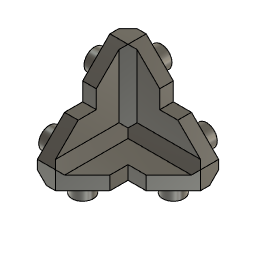
Frame_Corners v4 (Autodesk Fusion 360 design; units mm, degrees)
Autodesk Fusion 360 part; units mm, degrees
sketch "Sketch1" plane through (0, 0, 0) normal (0, 0, 1) x (1, 0, 0)
  circle A0 centre (0, 0) radius 2.5
  line L0 (0, 0) -> (1, 0)
  line L1 (1, 0) -> (11, 0)
  line L2 (0, 0) -> (0, -10)
  circle A1 centre (11, 0) radius 2.5
  circle A2 centre (0, -10) radius 2.5
  dimension "d1" = 5
  dimension "d2" = 10
  dimension "d3" = 10
  dimension "d4" = 5
  dimension "d5" = 5
  constraint coincident A0.centre L0.start
  constraint horizontal L0
  constraint parallel L0 L1
  constraint perpendicular L0 L2
  constraint coincident L1.end A1.centre
  constraint coincident L2.end A2.centre
  measures "d1" diameter of A0
  measures "d2" distance of L0.end L1.end
  measures "d3" distance of A0.centre L2.end
  measures "d4" diameter of A1
  measures "d5" diameter of A2
extrude "Extrude1" add sketch "Sketch1" along normal blind 2.5 makes body 1 at (2.4876, -9.7511, 1.6667) makes body 2 at (2.4876, -0.2489, 0.8333) makes body 3 at (13.4876, -0.2489, 0.8333)
sketch "Sketch2" plane through (0, 0, 2.5) normal (0, 0, 1) x (-1, 0, 0)
  circle A0 centre (0, 0) radius 2.5
  line L0 (0, 0) -> (0, -5)
  line L1 (0, 0) -> (5, 0)
  line L2 (0, 10) -> (0, 15)
  line L3 (5, 15) -> (-5, 15)
  line L4 (5, 15) -> (5, -5)
  line L5 (5, -5) -> (-15, -5)
  line L6 (-15, -5) -> (-15, 5)
  line L7 (-15, 5) -> (-5, 5)
  line L8 (-5, 5) -> (-5, 15)
  dimension "d8" = 5
  dimension "d9" = 5
  dimension "d10" = 5
  dimension "d11" = 10
  constraint coincident A0.centre L0.start
  constraint vertical L0
  constraint perpendicular L0 L1
  constraint vertical L2
  constraint horizontal L3
  constraint perpendicular L3 L4
  constraint perpendicular L4 L5
  constraint perpendicular L5 L6
  constraint perpendicular L6 L7
  measures "d8" distance of A0.centre L0.end
  measures "d9" distance of A0.centre L1.end
  measures "d10" distance of L2.start L2.end
  measures "d11" distance of L3.start L3.end
extrude "Extrude2" add sketch "Sketch2" along normal blind 3 contours A0 L0 L1 L4 L5 | A0 L0 L1 L3 L4 L5 L6 L7 L8 bodies 1 2 3
extrude "Extrude3" add 1 faces at (0.734, 0.5482, 2.5) along direction (0, 0, 1) blind 3 on bodies 1 bodies 1
sketch "Sketch3" plane through (0, 0, 5.5) normal (0, 0, 1) x (-1, 0, 0)
  line L0 (5, 15) -> (-5, 15)
  line L1 (-5, 15) -> (-5, 5)
  line L2 (-5, 5) -> (-15, 5)
  line L3 (-15, 5) -> (-15, -5)
  line L4 (-15, -5) -> (5, -5)
  line L5 (5, -5) -> (5, 15)
  line L6 (-15, -5) -> (-15, -2)
  line L7 (5, 15) -> (2, 15)
  line L8 (2, 15) -> (2, -2)
  line L9 (2, -2) -> (-15, -2)
  dimension "d16" = 3
  dimension "d17" = 3
  constraint coincident L3.end L4.start
  constraint perpendicular L4 L6
  constraint coincident L0.start L5.end
  constraint perpendicular L5 L7
  constraint perpendicular L7 L8
  measures "d16" distance of L3.end L6.end
  measures "d17" distance of L0.start L7.end
extrude "Extrude4" add sketch "Sketch3" along normal blind 17 contours L0 L3 L4 L5 L6 L7 L8 L9 bodies 1
sketch "Sketch4" plane through (0, 2, 0) normal (0, -1, 0) x (1, 0, 0)
  line L0 (-2, 5.5) -> (15, 5.5)
  line L1 (15, 5.5) -> (15, 22.5)
  line L2 (15, 22.5) -> (-2, 22.5)
  line L3 (-2, 22.5) -> (-2, 5.5)
  line L4 (15, 22.5) -> (15, 12.5)
  line L5 (15, 12.5) -> (5, 12.5)
  line L6 (5, 12.5) -> (5, 22.5)
  dimension "d20" = 10
  dimension "d21" = 10
  constraint coincident L1.end L2.start
  constraint perpendicular L2 L4
  constraint perpendicular L4 L5
  constraint coincident L2 L6.end
  constraint perpendicular L2 L6
  measures "d20" distance of L1.end L4.end
  measures "d21" distance of L4.end L5.end
extrude "Extrude5" cut sketch "Sketch4" against normal blind 3 contours L1 L2 L4 L5 L6 bodies 1
sketch "Sketch5" plane through (-2, 0, 0) normal (1, 0, 0) x (0, 1, 0)
  line L0 (-15, 5.5) -> (2, 5.5)
  line L1 (2, 5.5) -> (2, 22.5)
  line L2 (2, 22.5) -> (-15, 22.5)
  line L3 (-15, 22.5) -> (-15, 5.5)
  line L4 (-15, 22.5) -> (-5, 22.5)
  line L5 (-5, 22.5) -> (-5, 12.5)
  line L6 (-5, 12.5) -> (-15, 12.5)
  line L7 (-15, 12.5) -> (-15, 22.5)
  dimension "d24" = 10
  dimension "d25" = 10
  constraint horizontal L4
  constraint vertical L5
  constraint horizontal L6
  constraint vertical L7
  constraint coincident L2.end L3.start
  measures "d24" distance of L2.end L4.end
  measures "d25" distance of L2.end L6.end
extrude "Extrude6" cut sketch "Sketch5" against normal blind 3 contours L2 L3 L4 L5 L6 L7 bodies 1
sketch "Sketch6" plane through (-5, 0, 0) normal (-1, 0, 0) x (0, -1, 0)
  line L0 (15, 12.5) -> (5, 12.5)
  line L1 (5, 12.5) -> (5, 22.5)
  line L2 (5, 22.5) -> (-5, 22.5)
  line L3 (-5, 22.5) -> (-5, 2.5)
  line L4 (-5, 2.5) -> (15, 2.5)
  line L5 (15, 2.5) -> (15, 12.5)
  line L6 (0, 22.5) -> (0, 2.5)
  line L7 (15, 7) -> (-5, 7)
  circle A0 centre (0, 7) radius 2.5
  line L8 (0, 7) -> (10, 7)
  line L9 (0, 7) -> (0, 17)
  circle A1 centre (0, 17) radius 2.5
  circle A2 centre (10, 7) radius 2.5
  dimension "d28" = 5
  dimension "d29" = 10
  dimension "d30" = 10
  dimension "d31" = 5
  dimension "d32" = 5
  constraint midpoint L2 L6.start
  constraint coincident L4 L6.end
  constraint perpendicular L4 L6
  constraint coincident L5 L7.start
  constraint perpendicular L6 L7
  constraint coincident L6 A0.centre
  constraint coincident L7 A0.centre
  constraint coincident A0.centre L8.start
  constraint perpendicular L6 L8
  constraint perpendicular L7 L9
  constraint coincident L9.end A1.centre
  constraint coincident L8.end A2.centre
  measures "d28" diameter of A0
  measures "d29" distance of A0.centre L8.end
  measures "d30" distance of A0.centre L9.end
  measures "d31" diameter of A1
  measures "d32" diameter of A2
extrude "Extrude7" add sketch "Sketch6" along normal blind 2.5 contours L7 L8 A2 | L7 L8 A2 | L6 L9 A1 | L6 L9 A1 | L6 L7 A0 | L6 L7 A0 L8 | L6 L7 A0 L8 L9 | L6 L7 A0 L9 bodies 1
sketch "Sketch7" plane through (0, 5, 0) normal (0, 1, 0) x (-1, 0, 0)
  line L0 (-5, 12.5) -> (-15, 12.5)
  line L1 (-15, 12.5) -> (-15, 2.5)
  line L2 (-15, 2.5) -> (5, 2.5)
  line L3 (5, 2.5) -> (5, 22.5)
  line L4 (5, 22.5) -> (-5, 22.5)
  line L5 (-5, 22.5) -> (-5, 12.5)
  line L6 (0, 22.5) -> (0, 2.5)
  line L7 (-15, 7.5) -> (5, 7.5)
  circle A0 centre (0, 7.5) radius 2.5
  line L8 (0, 7.5) -> (0, 17.5)
  line L9 (0, 7.5) -> (-10, 7.5)
  circle A1 centre (-10, 7.5) radius 2.5
  circle A2 centre (0, 17.5) radius 2.5
  dimension "d35" = 5
  dimension "d36" = 10
  dimension "d37" = 10
  dimension "d38" = 5
  dimension "d39" = 5
  constraint midpoint L4 L6.start
  constraint coincident L2 L6.end
  constraint perpendicular L2 L6
  constraint midpoint L1 L7.start
  constraint coincident L3 L7.end
  constraint perpendicular L3 L7
  constraint coincident L6 A0.centre
  constraint coincident L7 A0.centre
  constraint coincident A0.centre L8.start
  constraint perpendicular L7 L8
  constraint perpendicular L6 L9
  constraint coincident L9.end A1.centre
  constraint coincident L8.end A2.centre
  measures "d35" diameter of A0
  measures "d36" distance of A0.centre L8.end
  measures "d37" distance of A0.centre L9.end
  measures "d38" diameter of A1
  measures "d39" diameter of A2
extrude "Extrude8" add sketch "Sketch7" along normal blind 2.5 contours L7 L9 A1 | L7 L9 A1 | L6 L8 A2 | L6 L8 A2 | L6 L7 A0 L9 | L6 L7 A0 | L6 L7 A0 L8 L9 | L6 L7 A0 L8 bodies 1
chamfer "Chamfer1" distance 2 angle 45 1 edges at (-5, 5, 12.5) on bodies 1
chamfer "Chamfer2" distance 2 angle 45 1 edges at (-5, -6, 2.5) on bodies 1
chamfer "Chamfer3" distance 2 angle 45 1 edges at (6, 5, 2.5) on bodies 1
chamfer "Chamfer4" distance 6 angle 45 1 edges at (15, 3.5, 12.5) on bodies 1
chamfer "Chamfer5" distance 6 angle 45 1 edges at (5, 3.5, 22.5) on bodies 1
chamfer "Chamfer6" distance 6 angle 45 1 edges at (-3.5, -5, 22.5) on bodies 1
chamfer "Chamfer7" distance 6 angle 45 1 edges at (-3.5, -15, 12.5) on bodies 1
chamfer "Chamfer8" distance 6 angle 45 1 edges at (5, -15, 4) on bodies 1
extrude "Extrude9" add 1 faces at (11.643, -0.1378, 0) along direction (0, 0, -1) blind 2.5 on bodies 1 bodies 1
extrude "Extrude10" cut 1 faces at (11.643, -0.1378, -2.5) along direction (0, 0, 1) blind 5 on bodies 1 bodies 1
sketch "Sketch8" plane through (0, 0, 2.5) normal (0, 0, -1) x (1, 0, 0)
  circle A0 centre (0, 10) radius 2.5
  circle A1 centre (0, 0) radius 2.5
  line L0 (5, 9) -> (-1, 15)
  line L1 (-1, 15) -> (-3, 15)
  line L2 (-3, 15) -> (-3, -3)
  line L3 (-3, -3) -> (15, -3)
  line L4 (15, -3) -> (15, 5)
  line L5 (15, 5) -> (5, 5)
  line L6 (5, 5) -> (5, 9)
  line L7 (0, 0) -> (10, 0)
  circle A2 centre (10, 0) radius 2.5
  dimension "d54" = 5
  constraint coincident A1.centre L7.start
  constraint horizontal L7
  constraint coincident L7.end A2.centre
  measures "d54" diameter of A2
extrude "Extrude11" add sketch "Sketch8" along normal blind 2.5 contours A2 bodies 1
chamfer "Chamfer9" distance 6 angle 45 1 edges at (15, -5, 4) on bodies 1
fillet "Fillet1" radius 0.5 1 edges at (12.3308, 7.5, 6.596) on bodies 1
fillet "Fillet3" radius 0.5 1 edges at (2.3308, 7.5, 16.596) on bodies 1
fillet "Fillet5" radius 0.5 1 edges at (-7.5, 2.3308, 16.096) on bodies 1
fillet "Fillet6" radius 0.5 1 edges at (-7.5, -7.6692, 6.096) on bodies 1
fillet "Fillet8" radius 0.5 1 edges at (7.6692, 0.904, 0) on bodies 1
fillet "Fillet9" radius 0.5 1 edges at (-2.3308, -10.904, 0) on bodies 1
chamfer "Chamfer10" distance 2 angle 45 1 edges at (-2, 2, 14) on bodies 1
chamfer "Chamfer11" distance 2 angle 45 1 edges at (7.5, 2, 5.5) on bodies 1
chamfer "Chamfer12" distance 2 angle 45 1 edges at (-2, -7.5, 5.5) on bodies 1
extrude "Extrude12" cut 1 faces at (-7.5, -0.4877, 7.5482) along direction (1, 0, 0) blind 2.5 on bodies 1 bodies 1
extrude "Extrude13" cut 1 faces at (0.5196, 7.5, 8.1515) along direction (0, -1, 0) blind 2.5 on bodies 1 bodies 1
extrude "Extrude14" cut 1 faces at (-0.7508, 0.3616, 0) along direction (0, 0, 1) blind 2.5 on bodies 1 bodies 1
sketch "Sketch9" plane through (0, 7.5, 0) normal (0, 1, 0) x (-1, 0, 0)
  circle A0 centre (-10, 7.5) radius 2
  circle A1 centre (-10, 7.5) radius 2.5
  circle A2 centre (-10, 7.5) radius 2.35
  dimension "d85" = 5
  dimension "d86" = 4.7
  constraint concentric A0 A1
  constraint concentric A1 A2
  measures "d85" diameter of A1
  measures "d86" diameter of A2
extrude "Extrude15" cut sketch "Sketch9" against normal blind 2.5 contours A1 bodies 1
sketch "Sketch10" plane through (0, 7.5, 0) normal (0, 1, 0) x (-1, 0, 0)
  circle A0 centre (0, 17.5) radius 2
  circle A1 centre (0, 17.5) radius 2.5
  circle A2 centre (0, 17.5) radius 2.35
  dimension "d89" = 5
  dimension "d90" = 4.7
  constraint concentric A0 A1
  constraint concentric A1 A2
  measures "d89" diameter of A1
  measures "d90" diameter of A2
extrude "Extrude16" cut sketch "Sketch10" against normal blind 2.5 contours A1 bodies 1
sketch "Sketch11" plane through (-7.5, 0, 0) normal (-1, 0, 0) x (0, -1, 0)
  circle A0 centre (0, 17) radius 2
  circle A1 centre (0, 17) radius 2.5
  circle A2 centre (0, 17) radius 2.35
  dimension "d93" = 5
  dimension "d94" = 4.7
  constraint concentric A0 A1
  constraint concentric A1 A2
  measures "d93" diameter of A1
  measures "d94" diameter of A2
extrude "Extrude17" cut sketch "Sketch11" against normal blind 2.5 contours A1 bodies 1
sketch "Sketch12" plane through (-7.5, 0, 0) normal (-1, 0, 0) x (0, -1, 0)
  circle A0 centre (10, 7) radius 2
  circle A1 centre (10, 7) radius 2.5
  circle A2 centre (10, 7) radius 2.35
  dimension "d97" = 5
  dimension "d98" = 4.7
  constraint concentric A0 A1
  constraint concentric A1 A2
  measures "d97" diameter of A1
  measures "d98" diameter of A2
extrude "Extrude18" cut sketch "Sketch12" against normal blind 2.5 contours A1 bodies 1
sketch "Sketch13" plane through (0, 0, 0) normal (0, 0, -1) x (1, 0, 0)
  circle A0 centre (0, 10) radius 2
  circle A1 centre (0, 10) radius 2.5
  circle A2 centre (0, 10) radius 2.35
  dimension "d101" = 5
  dimension "d102" = 4.7
  constraint concentric A0 A1
  constraint concentric A1 A2
  measures "d101" diameter of A1
  measures "d102" diameter of A2
extrude "Extrude19" cut sketch "Sketch13" against normal blind 2.5 contours A1 bodies 1
sketch "Sketch14" plane through (0, 0, 0) normal (0, 0, -1) x (1, 0, 0)
  circle A0 centre (10, 0) radius 2
  circle A1 centre (10, 0) radius 2.5
  circle A2 centre (10, 0) radius 2.35
  dimension "d105" = 5
  dimension "d106" = 4.7
  constraint concentric A0 A1
  constraint concentric A1 A2
  measures "d105" diameter of A1
  measures "d106" diameter of A2
extrude "Extrude20" cut sketch "Sketch14" against normal blind 2.5 contours A1 bodies 1
